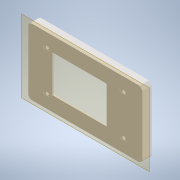
# Autodesk Inventor part: RPi Desk Case
Saved by Autodesk Inventor 2021 (Build 250183000, 183)
## iProperties
Created: 2022-06-16
Part Number: RPi Desk Case
Material: Generic
Document SubType Name: Modeling
Designer: cmzgt
Density: 1 g/cm^3
Appearance: Default
Author: cmzgt
Autodesk Inventor part; units mm, degrees
ref_plane "YZ Plane" through (0, 0, 0) normal (1, 0, 0) x (0, 1, 0)
ref_plane "XZ Plane" through (0, 0, 0) normal (0, 1, 0) x (-1, 0, 0)
ref_plane "XY Plane" through (0, 0, 0) normal (0, 0, 1) x (1, 0, 0)
ref_plane "Work Plane3" through (32.97, 21.365, 7.071) normal (0, 0, 1) x (1, 0, 0)
sketch "Sketch3" plane through (32.97, 21.365, 7.071) normal (0, 0, 1) x (1, 0, 0)
  line L0 (93.98, -54.61) -> (-93.98, -54.61)
  line L1 (-93.98, -54.61) -> (-93.98, 54.61)
  line L2 (-93.98, 54.61) -> (93.98, 54.61)
  line L3 (93.98, 54.61) -> (93.98, -54.61)
  line L4 (93.98, -54.61) -> (-93.98, 54.61) construction
  line L5 (-93.98, -54.61) -> (93.98, 54.61) construction
  line L6 (83.1, 48.8) -> (83.1, -50.3) projected
  line L7 (-81.6, 50.3) -> (81.6, 50.3) projected
  line L8 (32.5, 25) -> (32.5, -25) projected
  line L9 (-52.4242, -25) -> (-52.4242, 25) projected
  line L10 (-49.4242, 28) -> (29.5, 28) projected
  line L11 (29.5, -28) -> (-49.4242, -28) projected
  line L12 (35.04, -30.54) -> (-54.3292, -30.54)
  line L13 (-54.3292, -30.54) -> (-54.3292, 30.54)
  line L14 (-54.3292, 30.54) -> (35.04, 30.54)
  line L15 (35.04, 30.54) -> (35.04, -30.54)
  point P0 (-56.9284, 33.08)
  dimension "d6" = 187.96
  dimension "d7" = 109.22
  dimension "d8" = 4.31
  dimension "d9" = 10.88
  dimension "d51" = 1.905
  dimension "d52" = 2.54
  dimension "d53" = 2.54
  dimension "d54" = 2.54
  constraints: 20 end point, 4 parallel, 2 horizontal, 2 perpendicular, 1 point on line
  measures "d6" distance of L1.end L2.end
  measures "d7" distance of L0.end L1.end
  measures "d8" distance between parallel lines of L7 L2
  measures "d9" distance between parallel lines of L6 L3
  measures "d51" distance between parallel lines of L9 L13
  measures "d52" distance between parallel lines of L10 L14
  measures "d53" distance between parallel lines of L8 L15
  measures "d54" distance between parallel lines of L11 L12
extrude "Extrusion2" add sketch "Sketch3" against normal blind 2.54
sketch "Sketch5" plane through (32.97, 21.365, 7.071) normal (0, 0, 1) x (1, 0, 0)
  circle A0 centre (-63.1, 32.8) radius 1.5 projected
  circle A1 centre (-63.1, -32.8) radius 1.5 projected
  circle A2 centre (63.1, 32.8) radius 1.5 projected
  circle A3 centre (63.1, 32.8) radius 1.5 projected
  circle A4 centre (63.1, 32.8) radius 1.5 projected
  circle A5 centre (63.1, 32.8) radius 1.5 projected
  circle A6 centre (63.1, -32.8) radius 1.5 projected
  line L0 (-59.965, 36.77) -> (-59.965, 28.83) projected
  line L1 (-59.965, 36.77) -> (-66.235, 36.77) projected
  line L2 (-66.235, 36.77) -> (-66.235, 28.83) projected
  line L3 (-59.965, 28.83) -> (-66.235, 28.83) projected
  circle A7 centre (-63.1, 32.8) radius 1.5 projected
  line L4 (25.03, 27.635) -> (32.97, 27.635) projected
  line L5 (25.03, 27.635) -> (25.03, 21.365) projected
  line L6 (25.03, 21.365) -> (32.97, 21.365) projected
  line L7 (32.97, 27.635) -> (32.97, 21.365) projected
  circle A8 centre (29, 24.5) radius 1.25 projected
  line L8 (-59.965, -28.83) -> (-59.965, -36.77) projected
  line L9 (-59.965, -28.83) -> (-66.235, -28.83) projected
  line L10 (-66.235, -28.83) -> (-66.235, -36.77) projected
  line L11 (-59.965, -36.77) -> (-66.235, -36.77) projected
  circle A9 centre (-63.1, -32.8) radius 1.5 projected
  line L12 (66.235, -28.83) -> (66.235, -36.77) projected
  line L13 (66.235, -28.83) -> (59.965, -28.83) projected
  line L14 (59.965, -28.83) -> (59.965, -36.77) projected
  line L15 (66.235, -36.77) -> (59.965, -36.77) projected
  circle A10 centre (63.1, -32.8) radius 1.5 projected
  line L16 (66.235, 36.77) -> (66.235, 28.83) projected
  line L17 (66.235, 36.77) -> (59.965, 36.77) projected
  line L18 (59.965, 36.77) -> (59.965, 28.83) projected
  line L19 (66.235, 28.83) -> (59.965, 28.83) projected
  circle A11 centre (63.1, 32.8) radius 1.5 projected
  point P0 (-32.97, -21.365)
sketch "Sketch4" plane through (32.97, 21.365, 7.071) normal (0, 0, 1) x (1, 0, 0)
  circle A0 centre (-63.1, 32.8) radius 1.5 projected
  circle A1 centre (-63.1, -32.8) radius 1.5 projected
  circle A2 centre (63.1, -32.8) radius 1.5 projected
  circle A3 centre (63.1, 32.8) radius 1.5 projected
  circle A4 centre (-63.1, 32.8) radius 2.54
  circle A5 centre (63.1, 32.8) radius 2.54
  circle A6 centre (-63.1, -32.8) radius 2.54
  circle A7 centre (63.1, -32.8) radius 2.54
  point P0 (-32.97, -21.365)
  dimension "d12" = 5.08
  constraints: 4 centre point, 4 coincident, 3 equal radius
  measures "d12" diameter of A4
ref_plane "Work Plane4" through (92.935, -15.405, 0) normal (0, 0, 1) x (1, 0, 0)
extrude "Extrusion3" add sketch "Sketch5" against normal up to surface (7.071 mm away) contours A2 | A6 | L0 L3 L2 L1 | L8 L11 L10 L9 | L12 L15 L14 L13 | L16 L19 L18 L17
extrude "Extrusion4" cut sketch "Sketch4" against normal up to surface (7.071 mm away) contours A0 | A1 | A2 | A3 | A4 | A5 | A6 | A7
ref_plane "Work Plane5" through (-62.51, -33.015, -8.55) normal (0, 0, 1) x (1, 0, 0)
sketch "Sketch7" plane through (32.97, 21.365, 4.531) normal (0, 0, -1) x (-1, 0, 0)
  line L0 (-91.44, 52.07) -> (91.44, 52.07)
  line L1 (91.44, 52.07) -> (91.44, -52.07)
  line L2 (91.44, -52.07) -> (-91.44, -52.07)
  line L3 (-91.44, -52.07) -> (-91.44, 52.07)
  line L4 (-91.44, 52.07) -> (91.44, -52.07) construction
  line L5 (91.44, 52.07) -> (-91.44, -52.07) construction
  line L6 (-93.98, -54.61) -> (93.98, -54.61) projected
  line L7 (93.98, -54.61) -> (93.98, 54.61) projected
  line L8 (-93.98, 54.61) -> (-93.98, -54.61) projected
  line L9 (93.98, 54.61) -> (-93.98, 54.61) projected
  point P0 (32.97, -21.365)
  point P1 (0, 0)
  dimension "d22" = 2.54
  dimension "d23" = 2.54
  dimension "d24" = 2.54
  dimension "d25" = 2.54
  constraints: 12 end point, 2 midpoint, 2 parallel, 1 horizontal, 1 perpendicular
  measures "d22" distance between parallel lines of L6 L2
  measures "d23" distance between parallel lines of L7 L1
  measures "d24" distance between parallel lines of L8 L3
  measures "d25" distance between parallel lines of L9 L0
extrude "Extrusion5" add sketch "Sketch7" along normal up to surface (13.081 mm away)
fillet "Fillet1" radius 6.63 4 edges at (-61.01, 75.975, -0.7395) (126.95, 75.975, -0.7395) (126.95, -33.245, -0.7395) (-61.01, -33.245, -0.7395)
sketch "Sketch9" plane through (32.97, 21.365, 7.071) normal (0, 0, 1) x (1, 0, 0)
  circle A0 centre (-63.1, -32.8) radius 2.54 projected
  circle A1 centre (-63.1, 32.8) radius 2.54 projected
  circle A2 centre (63.1, 32.8) radius 2.54 projected
  line L0 (66.275, -32.8) -> (59.925, -32.8) construction
  circle A3 centre (63.1, -32.8) radius 2.54 projected
  line L1 (66.275, -29.625) -> (59.925, -29.625)
  line L2 (59.925, -35.975) -> (66.275, -35.975)
  arc A4 (66.275, -35.975) -> (66.275, -29.625) centre (66.275, -32.8) ccw
  arc A5 (59.925, -29.625) -> (59.925, -35.975) centre (59.925, -32.8) ccw
  line L3 (-59.925, -32.8) -> (-66.275, -32.8) construction
  line L4 (-59.925, -29.625) -> (-66.275, -29.625)
  line L5 (-66.275, -35.975) -> (-59.925, -35.975)
  arc A6 (-59.925, -35.975) -> (-59.925, -29.625) centre (-59.925, -32.8) ccw
  arc A7 (-66.275, -29.625) -> (-66.275, -35.975) centre (-66.275, -32.8) ccw
  line L6 (66.275, 32.8) -> (59.925, 32.8) construction
  line L7 (59.965, 36.77) -> (59.965, 28.83) projected
  line L8 (66.275, 35.975) -> (59.925, 35.975)
  line L9 (59.925, 29.625) -> (66.275, 29.625)
  arc A8 (66.275, 29.625) -> (66.275, 35.975) centre (66.275, 32.8) ccw
  arc A9 (59.925, 35.975) -> (59.925, 29.625) centre (59.925, 32.8) ccw
  line L10 (-59.925, 32.8) -> (-66.275, 32.8) construction
  line L11 (-59.925, 35.975) -> (-66.275, 35.975)
  line L12 (-66.275, 29.625) -> (-59.925, 29.625)
  arc A10 (-59.925, 29.625) -> (-59.925, 35.975) centre (-59.925, 32.8) ccw
  arc A11 (-66.275, 35.975) -> (-66.275, 29.625) centre (-66.275, 32.8) ccw
  point P0 (-32.97, -21.365)
  dimension "d47" = 3.175
  dimension "d48" = 6.35
  constraints: 32 end point, 16 point on circle, 16 tangent, 8 centre point, 4 midpoint, 4 parallel, 3 equal length, 3 equal radius, 2 point on line, 1 horizontal, 1 perpendicular
  measures "d47" distance of A3.centre L0.end
  measures "d48" diameter of A5
extrude "Extrusion6" cut sketch "Sketch9" against normal blind 0.381 contours A0 | A1 | A2 | A3 | A4 L2 A5 L1 | A6 L5 A7 L4 | L8 A8 L9 L7 | L7 L9 A9 L8 | A10 L12 A11 L11
body "Solid2"
